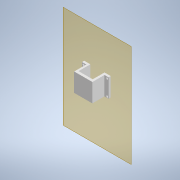
# Autodesk Inventor part: MotorLock
Saved by Autodesk Inventor 2021 (Build 250183000, 183)
## iProperties
Created: 2020-09-18
Part Number: MotorLock
Material: Generic
Document SubType Name: Modeling
Designer: siwat
Density: 1 g/cm^3
Appearance: Default
Author: siwat
Autodesk Inventor part; units mm, degrees
ref_plane "YZ Plane" through (0, 0, 0) normal (1, 0, 0) x (0, 1, 0)
ref_plane "XZ Plane" through (0, 0, 0) normal (0, 1, 0) x (-1, 0, 0)
ref_plane "XY Plane" through (0, 0, 0) normal (0, 0, 1) x (1, 0, 0)
ref_plane "Work Plane1" through (0, 0, 0) normal (0, 0, 1) x (1, 0, 0)
sketch "Sketch1" plane through (0, 0, 0) normal (0, 0, 1) x (1, 0, 0)
  line L0 (21.9816, 24.6798) -> (-20.9074, 24.6798)
  line L1 (-20.9074, 24.6798) -> (-20.9074, -5.2231)
  line L2 (-20.9074, -5.2231) -> (21.9816, -5.2231)
  line L3 (21.9816, -5.2231) -> (21.9816, 24.6798)
  line L4 (-10.9398, 24.6798) -> (-10.9398, -5.2231)
  line L5 (11.8882, 24.6798) -> (11.8882, -5.2231)
  circle A0 centre (19.7466, 22.1825) radius 1.5378
  circle A1 centre (19.7466, -3.0178) radius 1.5307
  circle A2 centre (-18.5031, -1.487) radius 1.5327
  circle A3 centre (-18.5031, 22.1825) radius 1.5785
  point P0 (0, 0)
  constraints: 12 end point, 4 centre point, 4 point on line, 3 perpendicular, 2 parallel, 1 horizontal
ref_plane "Work Plane2" through (0, 0, 0) normal (0, 0, 1) x (1, 0, 0)
extrude "Extrusion1" add sketch "Sketch1" along normal blind 3.65 contours L3 L2 L5 L0 | L4 L2 L1 L0
sketch "Sketch3" plane through (0, 0, 3.65) normal (0, 0, 1) x (1, 0, 0)
  line L0 (11.8882, 24.6798) -> (11.8882, -5.2231) projected
  line L1 (21.9816, 24.6798) -> (11.8882, 24.6798) projected
  line L2 (11.8882, -5.2231) -> (15.3769, -5.2231)
  line L3 (15.3769, -5.2231) -> (15.3769, 24.6798)
  line L4 (15.3769, 24.6798) -> (11.8882, 24.6798)
  line L5 (11.8882, 24.6798) -> (11.8882, -5.2231)
  line L6 (-10.9398, 24.6798) -> (-20.9074, 24.6798) projected
  line L7 (-10.9398, -5.2231) -> (-13.9699, -5.2231)
  line L8 (-13.9699, -5.2231) -> (-13.9699, 24.6798)
  line L9 (-13.9699, 24.6798) -> (-10.9398, 24.6798)
  line L10 (-10.9398, 24.6798) -> (-10.9398, -5.2231)
  point P0 (0, 0)
  constraints: 16 end point, 4 parallel, 2 horizontal, 2 perpendicular, 2 point on line
extrude "Extrusion2" add sketch "Sketch3" along normal blind 19.525
sketch "Sketch4" plane through (-10.9398, -5.2231, 0) normal (1, 0, 0) x (0, 0, -1)
  line L0 (0, 0) -> (-23.175, 0) projected
  line L1 (0, 29.9028) -> (-23.175, 29.9028) projected
  line L2 (-23.175, 0) -> (-19.0955, 0)
  line L3 (-19.0955, 0) -> (-19.0955, 29.9028)
  line L4 (-19.0955, 29.9028) -> (-23.175, 29.9028)
  line L5 (-23.175, 29.9028) -> (-23.175, 0)
  point P0 (0, 5.2231)
  constraints: 8 end point, 2 parallel, 1 horizontal, 1 perpendicular, 1 point on line
extrude "Extrusion3" add sketch "Sketch4" along normal up to surface (22.828 mm away)
body "Solid1"
